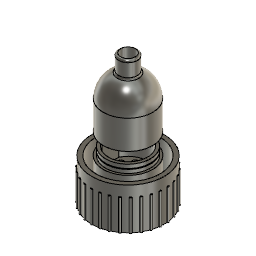
bw_charge_point (Autodesk Fusion 360 design; units mm, degrees)
part number: 2026-05-08-20-14-07-458
part number: 2026-05-08-20-40-07-463
part number: 2026-05-08-21-07-22-455
Autodesk Fusion 360 part; units mm, degrees
sketch "Sketch1" plane through (0, 0, 0) normal (0, 0, 1) x (1, 0, 0)
  circle A0 centre (0, 0) radius 15.4
  circle A1 centre (0, 0) radius 17.5
  dimension "d1" = 30.8
  dimension "d2" = 35
  constraint coincident A0.centre A1.centre
  constraint concentric A0 A1
  measures "d1" diameter of A0
  measures "d2" diameter of A1
extrude "Extrude1" add sketch "Sketch1" along normal blind 20 makes body 1
sketch "Sketch2" plane through (0, 0, 0) normal (0, 0, -1) x (1, 0, 0)
  circle A0 centre (0, 0) radius 15.4
  circle A1 centre (0, 0) radius 17.5
  line L0 (15, 2.5) -> (16, 2.5)
  line L1 (16, 2.5) -> (16, -2.5)
  line L2 (16, -2.5) -> (15, -2.5)
  line L3 (15, -2.5) -> (15, 2.5)
  constraint horizontal L0
  constraint vertical L1
  constraint horizontal L2
  constraint vertical L3
extrude "Extrude2" add sketch "Sketch2" against normal blind 10 separate body contours A0 L0 L2 L3 picked at (15.1258, -0.2789) makes body 2
sketch "Sketch3" plane through (15, 0, 0) normal (-1, 0, 0) x (0, -1, 0)
  line L0 (-2.5, 0) -> (2.5, 0)
  line L1 (2.5, 0) -> (2.5, 10)
  line L2 (2.5, 10) -> (-2.5, 10)
  line L3 (-2.5, 10) -> (-2.5, 0)
  circle A0 centre (0, 2.5) radius 2
  dimension "d7" = 4
  measures "d7" diameter of A0
extrude "Extrude3" add sketch "Sketch3" along normal blind 1 and the other way blind 1 separate body contours A0 makes body 3
delete_body "RemoveBody1" bodies 2
extrude "Extrude4" add 1 faces at (14, -0.4887, 2.5604) along direction (-1, 0, 0) blind 0.5 on bodies 3 bodies 3
extrude "Extrude5" cut 1 faces at (16, -0.4887, 2.5604) along direction (-1, 0, 0) blind 0.6 on bodies 3 bodies 1 3
fillet "Fillet1" radius 0.5 1 edges at (13.5, 1.8647, 1.7768) on bodies 3
pattern_circular "C-Pattern1" count 3 over 360 about axis through (0, 0, 1.75) along (0, 0, 1) of bodies 3 makes body 4 at (-5.7432, 13.9277, 2.3009) makes body 5 at (-9.1901, -11.9376, 2.3009)
sketch "Sketch4" plane through (0, 0, 0) normal (0, 0, -1) x (1, 0, 0)
  circle A0 centre (0, 0) radius 15.4
  circle A1 centre (0, 0) radius 17.5
  circle A2 centre (0, 17.5) radius 0.5
  dimension "d20" = 1
  constraint coincident A1 A2.centre
  measures "d20" diameter of A2
extrude "Extrude6" add sketch "Sketch4" against normal blind 15 separate body contours A1 A2 picked at (-0.0012, 17.6661) makes body 6
pattern_circular "C-Pattern2" count 30 over 360 about axis through (0, 0, 1.75) along (0, 0, 1) of bodies 6 makes body 7 at (4.1205, -17.2503, 10) makes body 8 at (6.6682, -16.2056, 10) makes body 9 at (9.8918, -14.4651, 10) makes body 10 at (12.6831, -12.0924, 10) makes body 11 at (14.9201, -9.1912, 10) makes body 12 at (16.505, -5.8882, 10) makes body 13 at (17.5112, -2.3177, 10) makes body 14 at (17.473, 1.334, 10) makes body 15 at (16.5119, 5.8902, 10) makes body 16 at (15.4198, 8.3256, 10) makes body 17 at (13.3519, 11.3496, 10) makes body 18 at (10.7362, 13.9397, 10) makes body 19 at (7.5812, 15.7991, 10) makes body 20 at (3.1781, 17.3126, 10) makes body 21 at (0.4997, 17.5168, 10) makes body 22 at (-4.0865, 17.3396, 10) makes body 23 at (-6.6682, 16.2056, 10) makes body 24 at (-9.8918, 14.4651, 10) makes body 25 at (-12.6831, 12.0924, 10) makes body 26 at (-14.9201, 9.1912, 10) makes body 27 at (-16.505, 5.8882, 10) makes body 28 at (-17.5112, 2.3177, 10) makes body 29 at (-17.473, -1.334, 10) makes body 30 at (-16.5119, -5.8902, 10) makes body 31 at (-15.4198, -8.3256, 10) makes body 32 at (-13.3519, -11.3496, 10) makes body 33 at (-10.7362, -13.9397, 10) makes body 34 at (-7.4626, -16.3492, 5) makes body 35 at (-3.1781, -17.3126, 10)
combine "Combine1" operation add target body 1 tool bodies 3 14 15 13 9 5 8 7 10 11 12 22 23 21 24 25 26 27 28 29 30 31 32 33 34 35 6 16 19 18 20 17 4
copy_body "Body->Comp1" bodies 1 removing the originals makes body 36 in component "lock_ring"
sketch "Sketch5" plane through (0, 0, 0) normal (0, 0, 1) x (1, 0, 0)
  circle A0 centre (0, 0) radius 9.4
  circle A1 centre (0, 0) radius 11.9
  dimension "d25" = 18.8
  dimension "d26" = 23.8
  constraint coincident A0.centre A1.centre
  constraint concentric A0 A1
  measures "d25" diameter of A0
  measures "d26" diameter of A1
extrude "Extrude7" add sketch "Sketch5" along normal blind 19 separate body makes body 37
sketch "Sketch6" plane through (0, 0, 19) normal (0, 0, 1) x (-1, 0, 0)
  circle A0 centre (0, 0) radius 9.4
  circle A1 centre (0, 0) radius 11.9
  circle A2 centre (0, 0) radius 9.5
  circle A3 centre (-2.4871, 6.0044) radius 1.3
  circle A4 centre (0, 0) radius 6.4991 construction
  circle A5 centre (-6.0044, 2.4871) radius 1.3
  circle A6 centre (-6.0044, -2.4871) radius 1.3
  circle A7 centre (-2.4871, -6.0044) radius 1.3
  circle A8 centre (2.4871, -6.0044) radius 1.3
  circle A9 centre (6.0044, -2.4871) radius 1.3
  circle A10 centre (6.0044, 2.4871) radius 1.3
  circle A11 centre (2.4871, 6.0044) radius 1.3
  line L0 (0, 0) -> (0, 1.6029) construction
  line L1 (-6.4991, 0) -> (6.4991, 0) construction
  circle A12 centre (-2.4, 0) radius 1.3
  circle A13 centre (2.4, 0) radius 1.3
  dimension "d33" = 2.6
  dimension "d36" = 360
  dimension "d37" = 2.6
  dimension "d38" = 2.6
  dimension "d39" = 4.8
  constraint coincident A0.centre A1.centre
  constraint coincident A3.centre A4
  constraint vertical L0
  constraint symmetric A3.centre A11.centre L0
  constraint coincident A4 L1.start
  constraint coincident A4 L1.end
  constraint horizontal L1
  constraint coincident L1 A12.centre
  constraint coincident L1 A13.centre
  constraint symmetric L0 A12.centre A13.centre
  measures "d33" diameter of A3
  measures "d37" diameter of A12
  measures "d38" diameter of A13
  measures "d39" distance of A12.centre A13.centre
extrude "Extrude8" add sketch "Sketch6" against normal blind 9 contours A0 | A2 | A3 | A5 | A6 | A7 | A8 | A9 | A10 | A11 | A12 | A13 bodies 37
sketch "Sketch7" plane through (0, 0, 19) normal (0, 0, 1) x (-1, 0, 0)
  circle A0 centre (0, 0) radius 11.9
  circle A1 centre (0, 0) radius 9.4
  dimension "d50" = 18.8
  constraint coincident A0.centre A1.centre
  measures "d50" diameter of A1
extrude "Extrude9" cut sketch "Sketch7" against normal blind 6 contours A1 bodies 37
extrude "Extrude10" cut sketch "Sketch6" against normal blind 10 contours A3 | A5 | A6 | A7 | A8 | A9 | A10 | A11 | A12 | A13 bodies 37
sketch "Sketch8" plane through (0, 0, 19) normal (0, 0, 1) x (-1, 0, 0)
  circle A0 centre (0, 0) radius 9.4
  circle A1 centre (0, 0) radius 11.9
  line L0 (9.1194, -1) -> (12.1194, -1)
  line L1 (12.1194, -1) -> (12.1194, 1)
  line L2 (12.1194, 1) -> (9.1194, 1)
  line L3 (9.1194, 1) -> (9.1194, -1)
  line L4 (0, 0) -> (13.2042, 0) construction
  dimension "d42" = 3
  dimension "d43" = 2
  constraint horizontal L0
  constraint vertical L1
  constraint horizontal L2
  constraint vertical L3
  constraint coincident A0.centre A1.centre
  constraint perpendicular L1 L4
  constraint symmetric L0 L2 L4
  measures "d42" distance of L0.start L0.end
  measures "d43" distance of L0.start L2.end
extrude "Extrude11" cut sketch "Sketch8" against normal blind 19 contours A0 A1 L0 L2 picked at (10.2172, -0.5561) bodies 37
copy_body "Body->Comp2" bodies 37 removing the originals makes body 38 in component "pin_body"
extrude "Extrude1'" add 1 faces at (11.0161, -0.8072, 19) along direction (0, 0, 1) blind 1 on bodies 38 bodies 38 in component "pin_body"
sketch "Sketch9" plane through (0, 0, 13) normal (0, 0, 1) x (-1, 0, 0)
  arc A0 (9.3467, 1) -> (9.3467, -1) centre (0, 0) ccw
  arc A1 (9.3467, -1) -> (9.3467, 1) centre (0, 0) ccw
  circle A2 centre (6.0044, -2.4871) radius 1.3
  circle A3 centre (-2.4, 0) radius 1.3
  circle A4 centre (-2.4871, 6.0044) radius 1.3
  circle A5 centre (2.4871, 6.0044) radius 1.3
  circle A6 centre (-6.0044, -2.4871) radius 1.3
  circle A7 centre (2.4871, -6.0044) radius 1.3
  circle A8 centre (2.4, 0) radius 1.3
  circle A9 centre (-6.0044, 2.4871) radius 1.3
  circle A10 centre (6.0044, 2.4871) radius 1.3
  circle A11 centre (-2.4871, -6.0044) radius 1.3
  line L0 (8.5018, 4.0099) -> (8.5018, -4.0099)
  constraint coincident A0 L0.start
  constraint coincident A0 L0.end
  constraint vertical L0
extrude "Extrude2'" add sketch "Sketch9" along normal blind 7 and the other way blind 13 contours A0 A1 L0 bodies 38 in component "pin_body"
sketch "Sketch10" plane through (0, 0, 20) normal (0, 0, 1) x (-1, 0, 0)
  line L0 (9.3467, 1) -> (11.8579, 1)
  arc A0 (11.8579, 1) -> (11.8579, -1) centre (0, 0) ccw
  line L1 (11.8579, -1) -> (9.3467, -1)
  arc A1 (9.3467, -1) -> (9.3467, 1) centre (0, 0) ccw
  line L2 (8.5018, 4.0099) -> (8.5018, -4.0099)
  arc A2 (8.5018, 4.0099) -> (8.5018, -4.0099) centre (0, 0) ccw
  circle A3 centre (0, 0) radius 11.9
  constraint concentric A0 A3
  constraint coincident A0.end A3
extrude "Extrude3'" add sketch "Sketch10" along normal blind 10 separate body makes body 39 in component "pin_body"
extrude "Extrude4'" add 1 faces at (-9.6345, 0, 20) along direction (0, 0, -1) blind 4 on bodies 39 bodies 39 in component "pin_body"
ref_plane "WorkPlane1" through (0, 0, 18) normal (0, 0, -1) x (1, 0, 0) in component "pin_body"
sketch "Sketch1 (2)" plane through (0, 0, 18) normal (0, 0, -1) x (-1, 0, 0) in component "pin_body"
sketch "Sketch2 (2)" plane through (0, 0, 16) normal (0, 0, -1) x (1, 0, 0) in component "pin_body"
  arc A0 (-8.5018, -4.0099) -> (-8.5018, 4.0099) centre (0, 0) ccw
  line L0 (-8.5018, -4.0099) -> (-8.5018, 4.0099)
  circle A1 centre (0, 0) radius 11.9
  arc A2 (-10.0018, -4.3329) -> (-10.0018, 4.3329) centre (0, 0) ccw
  line L1 (-10.0018, -4.3329) -> (-10.0018, 4.3329)
  dimension "d59" = -1.5
extrude "Extrude5'" cut sketch "Sketch2 (2)" against normal blind 4 contours A2 L1 bodies 39 in component "pin_body"
sketch "Sketch3 (2)" plane through (0, 0, 18) normal (0, 0, -1) x (-1, 0, 0) in component "pin_body"
  circle A0 centre (0, 0) radius 10.9
  circle A1 centre (0, 0) radius 3.5
  circle A2 centre (0, 0) radius 4.5
  dimension "d62" = 21.8
  dimension "d80" = 7
  dimension "d81" = 9
  constraint coincident A0.centre A1.centre
  constraint concentric A0 A2
  measures "d62" diameter of A0
  measures "d80" diameter of A1
  measures "d81" diameter of A2
torus "TorusPrimitive1" add centre line diameter 21.932 section diameter 0.5 placed x (-1, 0, 0) y (0, 1, 0) z (0, 0, -1) at (0, 0, 18) bodies 39 in component "pin_body"
move_body "Move1" bodies 39 to x (1, 0, 0) y (0, 1, 0) z (0, 0, 1) at (0, 0, 12) in component "pin_body"
extrude "Extrude6'" cut 1 faces at (-10.6345, 0, 28) along direction (0, 0, 1) blind 0.1 on bodies 39 bodies 39 in component "pin_body"
move_body "Move2" bodies 39 to x (1, 0, 0) y (0, 1, 0) z (0, 0, 1) at (0, 0, -12) in component "pin_body"
move_body "Move3" bodies 39 to x (1, 0, 0) y (0, 1, 0) z (0, 0, 1) at (0, 0, 34) in component "pin_body"
extrude "Extrude7'" add 1 faces at (-9.8087, -2.5869, 20) along direction (0, 0, 1) blind 4 on bodies 38 bodies 38 in component "pin_body"
move_body "Move4" bodies 39 to x (1, 0, 0) y (0, 1, 0) z (0, 0, 1) at (0, 0, -30) in component "pin_body"
combine "Combine1'" operation cut target body 38 tool bodies 39 keep tools in component "pin_body"
move_body "Move5" bodies 39 to x (1, 0, 0) y (0, 1, 0) z (0, 0, 1) at (0, 0, 10) in component "pin_body"
sketch "Sketch5 (2)" plane through (0, 0, 24) normal (0, 0, 1) x (-1, 0, 0) in component "pin_body"
  line L0 (8.5018, 4.0099) -> (8.5018, -4.0099)
  arc A0 (8.5018, 4.0099) -> (8.5018, -4.0099) centre (0, 0) ccw
  line L1 (10.0018, 1) -> (10.0018, 4.3329)
  arc A1 (10.0018, 4.3329) -> (10.0018, -4.3329) centre (0, 0) ccw
  line L2 (10.0018, -4.3329) -> (10.0018, -1)
  line L3 (10.0018, -1) -> (9.3467, -1)
  arc A2 (9.3467, -1) -> (9.3467, 1) centre (0, 0) ccw
  line L4 (9.3467, 1) -> (10.0018, 1)
  line L5 (9.9018, -4.3121) -> (9.9018, -1.1)
  line L6 (9.9018, -1.1) -> (9.2347, -1.1)
  arc A3 (9.2347, -1.1) -> (9.2347, 1.1) centre (0, 0) ccw
  line L7 (9.2347, 1.1) -> (9.9018, 1.1)
  line L8 (9.9018, 1.1) -> (9.9018, 4.3121)
  arc A4 (9.9018, 4.3121) -> (9.9018, -4.3121) centre (0, 0) ccw
  dimension "d69" = -0.1
extrude "Extrude8'" cut sketch "Sketch5 (2)" against normal blind 3.9 contours L1 A1 L2 L3 A2 L4 bodies 38 in component "pin_body"
extrude "Extrude9'" add 1 faces at (-9.4571, -1.1, 22.7) along direction (0, 1, 0) blind 2.5 on bodies 38 bodies 38 in component "pin_body"
ref_plane "WorkPlane2" through (0, 0, 44) normal (0, 0, 1) x (-1, 0, 0) in component "pin_body"
sphere "SpherePrimitive1" add diameter 23.8 placed x (1, 0, 0) y (0, 1, 0) z (0, 0, 1) at (0, 0, 44) separate body makes body 40 in component "pin_body"
split "Split1" by plane through (0, 0, 44) normal (0, 0, 1) bodies 40 makes body 41 at (-5.8991, -10.2175, 45.5533) in component "pin_body"
delete_body "RemoveBody1'" bodies 40 in component "pin_body"
sphere "SpherePrimitive2" cut diameter 22 placed x (1, 0, 0) y (0, -1, 0) z (0, 0, -1) at (0, 0, 44) bodies 41 in component "pin_body"
sketch "Sketch8 (2)" plane through (0, 0, 0) normal (0, 0, 1) x (1, 0, 0) in component "pin_body"
  circle A0 centre (0, 0) radius 3.5
  dimension "d77" = 7
  constraint coincident A0.centre origin
  measures "d77" diameter of A0
extrude "Extrude10'" cut sketch "Sketch8 (2)" along normal blind 66 bodies 41 in component "pin_body"
extrude "Extrude11'" add sketch "Sketch3 (2)" against normal blind 45 separate body contours A2 makes body 42 in component "pin_body"
extrude "Extrude12" cut 1 faces at (-4.1369, -0.3974, 18) along direction (0, 0, 1) blind 36 on bodies 42 bodies 42 in component "pin_body"
combine "Combine2" operation add target body 39 tool bodies 41 42 in component "pin_body"
fillet "Fillet1'" radius 3 1 edges at (3.2631, -1.2657, 54) on bodies 39 in component "pin_body"
fillet "Fillet2" radius 1 1 edges at (4.1955, -1.6273, 55.0164) on bodies 39 in component "pin_body"
fillet "Fillet3" radius 1 1 edges at (4.1955, 1.6273, 63) on bodies 39 in component "pin_body"
component "lock_ring" placed x (1, 0, 0) y (0, 1, 0) z (0, 0, 1) at (0, 0, 0)
component "pin_body" placed x (1, 0, 0) y (0, 1, 0) z (0, 0, 1) at (0, 0, 0)
